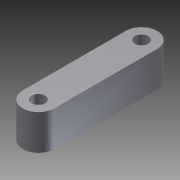
# Autodesk Inventor part: F
Saved by Autodesk Inventor 2011 SP2 (Build 150309200, 309)
## iProperties
Created: 2014-05-09
Part Number: F
Document SubType Name: Modeling
Designer: Maurice Woods
Density: 1 g/cm^3
Author: Maurice Woods
Autodesk Inventor part; units mm, degrees
ref_plane "YZ Plane" through (0, 0, 0) normal (1, 0, 0) x (0, 1, 0)
ref_plane "XZ Plane" through (0, 0, 0) normal (0, 1, 0) x (-1, 0, 0)
ref_plane "XY Plane" through (0, 0, 0) normal (0, 0, 1) x (1, 0, 0)
sketch "Sketch1" plane through (0, 0, 0) normal (0, 0, 1) x (1, 0, 0)
  line L0 (0, 17.1679) -> (0, 17.1679)
  line L1 (4, 13.1679) -> (4, -13.1679)
  line L2 (0, -17.1679) -> (0, -17.1679)
  line L3 (-4, -13.1679) -> (-4, 13.1679)
  line L4 (-4, 17.1679) -> (0, 17.1679) construction
  line L5 (0, 17.1679) -> (0, 0) construction
  line L6 (0, 0) -> (-4, 0) construction
  line L7 (-4, 0) -> (-4, 17.1679) construction
  arc A0 (4, 13.1679) -> (0, 17.1679) centre (0, 13.1679) ccw
  arc A1 (0, 17.1679) -> (-4, 13.1679) centre (0, 13.1679) ccw
  arc A2 (-4, -13.1679) -> (0, -17.1679) centre (0, -13.1679) ccw
  arc A3 (0, -17.1679) -> (4, -13.1679) centre (0, -13.1679) ccw
  dimension "d0" = 4
  dimension "d6" = 26.3358
  constraints: 16 end point, 8 point on circle, 8 tangent, 4 centre point, 4 parallel, 3 equal radius, 2 coincident, 2 horizontal, 2 perpendicular, 2 point on line, 2 other
  measures "d0" radius of A0
  measures "d6" distance of A2.centre A0.centre
extrude "Extrusion1" add sketch "Sketch1" along normal mid plane 9
sketch "Sketch2" plane through (0, 0, 4.5) normal (0, 0, 1) x (1, 0, 0)
  arc A0 (4, 13.1679) -> (-4, 13.1679) centre (0, 13.1679) ccw construction
  arc A1 (-4, -13.1679) -> (4, -13.1679) centre (0, -13.1679) ccw construction
  point P0 (0, 0)
hole "Hole1" at (0, 13.1679, 4.5) at (0, -13.1679, 4.5) direction (0, 0, -1) diameter 3.4 end through all clearance for "Socket Head Cap Screw" size "M3" standard "Ansi Metric M Profile"
equation "\"d6\" = LengthF"
equation "\"LengthF\" = 26.335787"
body "Solid1"
